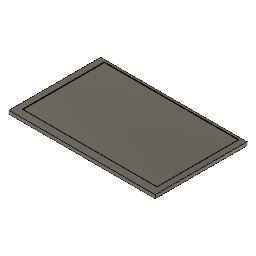
1680 5in TFT Display (Autodesk Fusion 360 design; units mm, degrees)
Autodesk Fusion 360 part; units mm, degrees
sketch "Sketch1" plane through (0, 0, 0) normal (0, 0, 1) x (1, 0, 0)
  line L0 (0, 0) -> (120.7, 0)
  line L1 (120.7, 0) -> (120.7, 75.8)
  line L2 (120.7, 75.8) -> (0, 75.8)
  line L3 (0, 75.8) -> (0, 0)
  line L4 (5, 73.8) -> (115.7, 73.8)
  line L5 (115.7, 73.8) -> (115.7, 6.4)
  line L6 (115.7, 6.4) -> (5, 6.4)
  line L7 (5, 6.4) -> (5, 73.8)
  dimension "d1" = 120.7
  dimension "d2" = 75.8
  dimension "d3" = 2
  dimension "d4" = 6.4
  dimension "d5" = 5
  dimension "d6" = 5
  measures "d1" distance of L1.end L2.end
  measures "d2" distance of L0.end L1.end
  measures "d3" distance of L2 L4
  measures "d4" distance of L0 L6
  measures "d5" distance of L1 L5
  measures "d6" distance of L3 L7
extrude "Extrude1" add sketch "Sketch1" along normal blind 3 contours L0 L1 L2 L3 | L4 L5 L6 L7
extrude "Extrude2" cut sketch "Sketch1" along normal blind 0.5 from surface at 2.5 contours L4 L5 L6 L7
